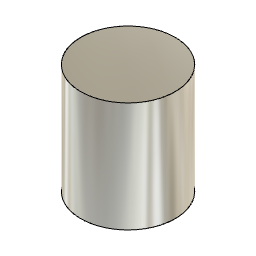
Center Pin (Autodesk Fusion 360 design; units mm, degrees)
Autodesk Fusion 360 part; units mm, degrees
sketch "Sketch1" plane through (0, 0, 0) normal (0, 0, 1) x (1, 0, 0)
  circle A0 centre (0, 0) radius 15
  dimension "d1" = 30
  constraint coincident A0.centre origin
  measures "d1" diameter of A0
extrude "Extrude1" add sketch "Sketch1" along normal blind 35
equation "d1 = Diameter / 5"
equation "Diameter = 150 mm"
equation "Thickness = 35 mm"
equation "d4 = Thickness"
equation "WaveAmplitude = 5 mm"
equation "WaveLength = 5"
